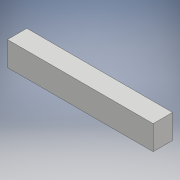
# Autodesk Inventor part: upor razyoma
Saved by Autodesk Inventor 2018.2 (Build 222227000, 227)
## iProperties
Created: 2026-01-20
Part Number: upor razyoma
Material: Типовые
Document SubType Name: Modeling
Designer: Denis
Density: 1 g/cm^3
Appearance: По умолчанию
Author: Denis
Autodesk Inventor part; units mm, degrees
ref_plane "YZ Plane" through (0, 0, 0) normal (1, 0, 0) x (0, 1, 0)
ref_plane "XZ Plane" through (0, 0, 0) normal (0, 1, 0) x (-1, 0, 0)
ref_plane "XY Plane" through (0, 0, 0) normal (0, 0, 1) x (1, 0, 0)
sketch "Эскиз1" plane through (0, 0, 0) normal (0, 0, 1) x (1, 0, 0)
  line L0 (0, 0) -> (12, 0)
  line L1 (12, 0) -> (12, -1.6)
  line L2 (12, -1.6) -> (0, -1.6)
  line L3 (0, -1.6) -> (0, 0)
  dimension "d0" = 12
  dimension "d1" = 1.6
  constraints: 8 end point, 2 parallel, 1 horizontal, 1 perpendicular
  measures "d0" distance of L1.end L2.end
  measures "d1" distance of L0.end L1.end
extrude "Выдавливание1" add sketch "Эскиз1" along normal blind 2
